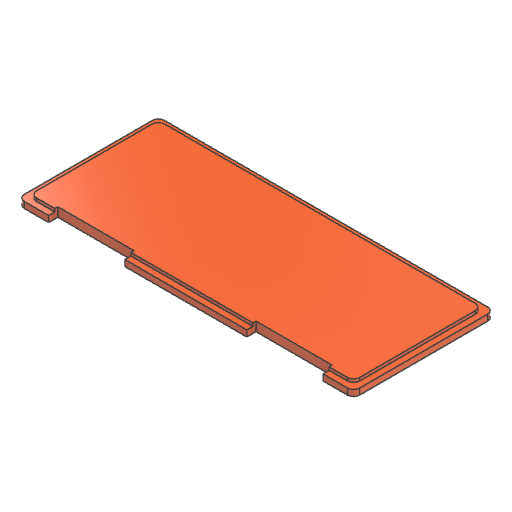
# Autodesk Inventor part: StereoPiBracketLidM12
Saved by Autodesk Inventor 2025.2 (Build 292293000, 293)
## iProperties
Created: 2024-08-20
Part Number: StereoPiBracketLidM12
Material: Generic
Document SubType Name: Modeling
Designer: 16366081
Density: 1 g/cm^3
Appearance: Default
Author: 16366081
Autodesk Inventor part; units mm, degrees
ref_plane "YZ Plane" through (0, 0, 0) normal (1, 0, 0) x (0, 1, 0)
ref_plane "XZ Plane" through (0, 0, 0) normal (0, 1, 0) x (-1, 0, 0)
sketch "Sketch1" plane through (0, 0, 0) normal (0, 1, 0) x (-1, 0, 0)
  line L0 (55, 23) -> (-55, 23)
  line L1 (-55, 23) -> (-55, -23)
  line L2 (-55, -23) -> (55, -23)
  line L3 (55, -23) -> (55, 23)
  line L4 (55, 23) -> (-55, -23) construction
  line L5 (-55, 23) -> (55, -23) construction
  point P0 (0, 0)
  point P1 (55, -4)
  point P2 (-55, -4)
  dimension "d0" = 110
  dimension "d1" = 46
  constraints: 12 end point, 2 midpoint, 2 parallel, 2 point on line, 1 horizontal, 1 perpendicular
  measures "d0" distance of L2.end L1.end
  measures "d1" distance of L1.end L0.end
extrude "Extrusion1" add sketch "Sketch1" along normal blind 2
sketch "Sketch2" plane through (0, 2, 0) normal (0, 1, 0) x (1, 0, 0)
  line L0 (-53, -21) -> (53, -21)
  line L1 (53, -21) -> (53, 21)
  line L2 (53, 21) -> (-53, 21)
  line L3 (-53, 21) -> (-53, -21)
  line L4 (-53, -21) -> (53, 21) construction
  line L5 (53, -21) -> (-53, 21) construction
  point P0 (0, 0)
  dimension "d14" = 106
  dimension "d15" = 42
  constraints: 12 end point, 2 midpoint, 2 parallel, 1 horizontal, 1 perpendicular
  measures "d14" distance of L2.end L1.end
  measures "d15" distance of L1.end L0.end
extrude "Extrusion2" add sketch "Sketch2" along normal blind 1
fillet "Fillet1" radius 2 8 edges at (53, 2.5, 21) (55, 1, 23) (55, 1, -23) (53, 2.5, -21) (-55, 1, -23) (-53, 2.5, -21) (-53, 2.5, 21) (-55, 1, 23)
sketch "Sketch3" plane through (0, 0, 0) normal (0, -1, 0) x (1, 0, 0)
  line L0 (-53, 23) -> (53, 23) projected
  line L1 (-45, 23) -> (-20, 23)
  line L2 (-20, 23) -> (-20, 20)
  line L3 (-20, 20) -> (-45, 20)
  line L4 (-45, 20) -> (-45, 23)
  line L5 (20, 23) -> (45, 23)
  line L6 (45, 23) -> (45, 20)
  line L7 (45, 20) -> (20, 20)
  line L8 (20, 20) -> (20, 23)
  line L9 (-55, -21) -> (-55, 21) projected
  line L10 (55, 21) -> (55, -21) projected
  point P0 (0, 0)
  point P1 (-55, 6)
  point P2 (-45, 21.5)
  point P3 (55, 6)
  point P4 (45, 21.5)
  dimension "d19" = 25
  dimension "d20" = 3
  dimension "d21" = 25
  dimension "d22" = 3
  dimension "d23" = 10
  dimension "d24" = 10
  constraints: 16 end point, 4 parallel, 2 horizontal, 2 midpoint, 2 perpendicular, 2 point on line
  measures "d19" distance of L2.end L3.end
  measures "d20" distance of L1.end L2.end
  measures "d21" distance of L6.end L7.end
  measures "d22" distance of L5.end L6.end
  measures "d23" distance from line of L9 point (-45, 21.5)
  measures "d24" distance from line of L10 point (45, 21.5)
extrude "Extrusion3" cut sketch "Sketch3" against normal through all
ref_plane "Work Plane2" through (0, 2, -23) normal (-1, 0, 0) x (0, -1, 0)
body "Solid1"
